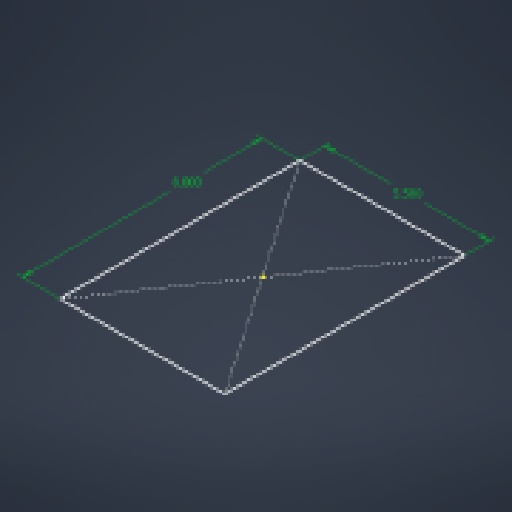
# Autodesk Inventor part: PLATE,KICKER,INSIDE
Saved by Autodesk Inventor 2026 (Build 300175000, 175)
## iProperties
Created: 2026-02-08
Part Number: PLATE,KICKER,INSIDE
Material: Aluminum 6061
Document SubType Name: Sheet Metal
Designer: littl
Density: 2.7 g/cm^3
Sheet Metal Rule: Default
Appearance: Aluminum - Flat
Author: littl
Autodesk Inventor part; units mm, degrees
ref_plane "YZ Plane" through (0, 0, 0) normal (1, 0, 0) x (0, 1, 0)
ref_plane "XZ Plane" through (0, 0, 0) normal (0, 1, 0) x (-1, 0, 0)
ref_plane "XY Plane" through (0, 0, 0) normal (0, 0, 1) x (1, 0, 0)
sketch "Sketch1" plane through (0, 0, 0) normal (0, 1, 0) x (-1, 0, 0)
  line L0 (-95.25, 101.6) -> (95.25, 101.6)
  line L1 (95.25, 101.6) -> (95.25, -101.6)
  line L2 (95.25, -101.6) -> (-95.25, -101.6)
  line L3 (-95.25, 101.6) -> (95.25, -101.6) construction
  line L4 (95.25, 101.6) -> (-95.25, -101.6) construction
  line L5 (-95.25, 101.6) -> (-184.15, 101.6)
  line L6 (-184.15, 101.6) -> (-184.15, 50.8)
  line L7 (-184.15, 50.8) -> (-95.25, 50.8)
  line L8 (-95.25, 50.8) -> (-95.25, 101.6) construction
  circle A0 centre (-142.1765, 70.739) radius 14.2875 construction
  line L9 (-95.25, 50.8) -> (-95.25, -101.6)
  circle A1 centre (-142.1765, 70.739) radius 25.4
  circle A2 centre (63.5, -44.5175) radius 14.2875 construction
  line L10 (45.5395, -26.557) -> (63.5, -44.5175) construction
  point P0 (0, 0)
  point P1 (55.8339, 70.739)
  point P2 (57.15, -92.075)
  point P3 (69.85, -92.075)
  point P4 (82.55, -92.075)
  point P5 (-43.7515, -91.186)
  point P6 (-2.4765, -62.611)
  point P7 (22.9235, -14.986)
  point P8 (-82.55, -92.075)
  point P9 (-69.85, -92.075)
  point P10 (-126.4413, 50.8)
  point P11 (-157.9117, 50.8)
  point P12 (45.5395, -62.478)
  point P13 (81.4605, -62.478)
  point P14 (81.4605, -26.557)
  dimension "d0" = 190.5
  dimension "d1" = 203.2
  dimension "d2" = 279.4
  dimension "d3" = 152.4
  dimension "d5" = 28.575
  dimension "d6" = 172.339
  dimension "d8" = 41.9735
  dimension "d9" = 198.0104
  dimension "d10" = 12.7
  dimension "d11" = 12.7
  dimension "d12" = 12.7
  dimension "d13" = 9.525
  dimension "d14" = 161.925
  dimension "d15" = 85.725
  dimension "d16" = 165.1
  dimension "d17" = 133.35
  dimension "d18" = 139.7
  dimension "d19" = 98.425
  dimension "d35" = 12.7
  dimension "d36" = 12.7
  dimension "d38" = 50.8
  dimension "d66" = 28.575
  dimension "d68" = 115.5112
  dimension "d69" = 25.4
  dimension "d70" = 45
  dimension "d73" = 360
  dimension "d75" = 31.75
  constraints: 22 end point, 5 horizontal alignment, 3 centre point, 3 coincident, 3 parallel, 3 perpendicular, 2 horizontal, 2 midpoint, 5 other
  measures "d0" distance of L1.end L2.end
  measures "d1" distance of L0.end L1.end
  measures "d2" distance between parallel lines of L1 L6
  measures "d3" distance between parallel lines of L2 L7
  measures "d5" diameter of A0
  measures "d6" distance from line of L2 point (-142.176, 70.739)
  measures "d8" distance from line of L6 point (-142.176, 70.739)
  measures "d9" distance of point (-142.176, 70.739) point (55.834, 70.739)
  measures "d10" distance from line of L1 point (82.55, -92.075)
  measures "d11" distance of point (69.85, -92.075) point (82.55, -92.075)
  measures "d12" distance of point (57.15, -92.075) point (69.85, -92.075)
  measures "d13" distance from line of L2 point (82.55, -92.075)
  measures "d14" vertical distance of point (-142.176, 70.739) point (-43.752, -91.186)
  measures "d15" vertical distance of point (-142.176, 70.739) point (22.923, -14.986)
  measures "d16" horizontal distance of point (-142.176, 70.739) point (22.923, -14.986)
  measures "d17" vertical distance of point (-142.176, 70.739) point (-2.477, -62.611)
  measures "d18" horizontal distance of point (-142.176, 70.739) point (-2.477, -62.611)
  measures "d19" horizontal distance of point (-142.176, 70.739) point (-43.752, -91.186)
  measures "d35" distance of point (-69.85, -92.075) point (-82.55, -92.075)
  measures "d36" distance from line of L9 point (-82.55, -92.075)
  measures "d38" diameter of A1
  measures "d66" diameter of A2
  measures "d68" distance of L10.end point (55.834, 70.739)
  measures "d69" distance of L10.end L10.start
  measures "d70" angle of L2 L10
  measures "d75" distance from line of L1 L10.end
extrude "Plate1" add sketch "Sketch1" along normal blind 4.7625
hole "Hole1" at (-57.15, 0, -92.075) at (-69.85, 0, -92.075) at (-82.55, 0, -92.075) at (43.7515, 0, -91.186) at (2.4765, 0, -62.611) at (-22.9235, 0, -14.986) at (82.55, 0, -92.075) at (69.85, 0, -92.075) at (-81.4605, 0, -62.478) at (-45.5395, 0, -26.557) at (-45.5395, 0, -62.478) at (-81.4605, 0, -26.557) direction (0, 1, 0) diameter 4.9784 depth 4.7625 tip angle 118 clearance for "Flat Head Machine Screw (82)" size "#10" standard "Ansi Unified Screw Threads"
hole "Hole2" at (142.1765, 0, 70.739) at (-55.8339, 0, 70.739) at (-63.5, 0, -44.5175) direction (0, 1, 0) diameter 28.575 depth 4.7625 tip angle 118
fillet "Corner Round1" radius 6.35 8 edges at (-95.25, 2.3813, 101.6) (184.15, 2.3813, 101.6) (184.15, 2.3813, 50.8) (95.25, 2.3813, 50.8) (-95.25, 2.3813, -101.6) (95.25, 2.3813, -101.6) (126.4413, 2.3813, 50.8) (157.9117, 2.3813, 50.8)
sketch "Sketch2" plane through (0, 4.7625, 0) normal (0, 1, 0) x (1, 0, 0)
  line L0 (184.15, -57.15) -> (184.15, -95.25) projected
  line L1 (-95.25, -95.25) -> (-95.25, 95.25) projected
  line L2 (177.8, -101.6) -> (-88.9, -101.6) projected
  point P0 (0, 0)
  point P1 (-88.9, -95.25)
  point P2 (25.4, -95.25)
  point P3 (38.1, -95.25)
  point P4 (50.8, -95.25)
  point P5 (177.2154, -95.25)
  dimension "d39" = 6.9346
  dimension "d40" = 6.35
  dimension "d41" = 6.35
  dimension "d43" = 12.7
  dimension "d44" = 12.7
  dimension "d52" = 114.3
  constraints: 4 horizontal alignment
  measures "d39" distance from line of L0 point (177.215, -95.25)
  measures "d40" distance from line of L1 point (-88.9, -95.25)
  measures "d41" distance from line of L2 point (-88.9, -95.25)
  measures "d43" distance of point (25.4, -95.25) point (38.1, -95.25)
  measures "d44" distance of point (38.1, -95.25) point (50.8, -95.25)
  measures "d52" distance of point (25.4, -95.25) point (-88.9, -95.25)
hole "Hole3" at (-88.9, 4.7625, 95.25) at (25.4, 4.7625, 95.25) at (38.1, 4.7625, 95.25) at (50.8, 4.7625, 95.25) at (177.2154, 4.7625, 95.25) direction (0, -1, 0) diameter 4.9784 depth 4.7625 tip angle 118 clearance for "Flat Head Machine Screw (82)" size "#10" standard "Ansi Unified Screw Threads"
sketch "Sketch3" plane through (0, 4.7625, 0) normal (0, 1, 0) x (1, 0, 0)
  line L0 (95.25, 95.25) -> (95.25, -44.45) projected
  line L1 (177.8, -101.6) -> (-88.9, -101.6) projected
  line L2 (184.15, -57.15) -> (184.15, -95.25) projected
  circle A0 centre (142.1765, -70.739) radius 14.2875 projected
  line L3 (142.1765, -70.739) -> (142.1765, -95.25) construction
  point P0 (0, 0)
  point P1 (170.7515, -63.5)
  point P2 (113.6015, -63.5)
  point P3 (82.55, -38.1)
  point P4 (82.55, -12.7)
  dimension "d53" = 25.4
  dimension "d54" = 57.15
  dimension "d55" = 12.7
  dimension "d56" = 63.5
  dimension "d58" = 38.1
  constraints: 2 end point, 1 horizontal alignment, 1 symmetric about line, 1 vertical, 1 vertical alignment
  measures "d53" distance of point (82.55, -38.1) point (82.55, -12.7)
  measures "d54" distance of point (170.752, -63.5) point (113.602, -63.5)
  measures "d55" distance from line of L0 point (82.55, -12.7)
  measures "d56" distance from line of L1 point (82.55, -38.1)
  measures "d58" distance from line of point (170.752, -63.5) L1
hole "Hole4" at (170.7515, 4.7625, 63.5) at (113.6015, 4.7625, 63.5) at (82.55, 4.7625, 38.1) at (82.55, 4.7625, 12.7) direction (0, -1, 0) diameter 4.9784 depth 4.7625 tip angle 118 clearance for "Flat Head Machine Screw (82)" size "#10" standard "Ansi Unified Screw Threads"
equation "\"d11\" = d10"
equation "\"d12\" = d10"
equation "\"d26\" = Thickness"
equation "\"d33\" = Thickness"
equation "\"d44\" = d43"
equation "\"d50\" = Thickness"
equation "\"d64\" = Thickness"
equation "\"d20\" = Thickness"
equation "\"BendRadius\" = Thickness"
equation "\"BendReliefWidth\" = Thickness"
equation "\"BendReliefDepth\" = 0.5 * Thickness"
equation "\"CornerReliefSize\" = 4 * Thickness"
equation "\"MinimumRemnant\" = 2 * Thickness"
equation "\"TransitionRadius\" = BendRadius"
equation "\"JacobiRadiusSize\" = BendRadius"
equation "\"GapSize\" = Thickness"
equation "\"Thickness\" = 4.7625"
body "Solid1"
